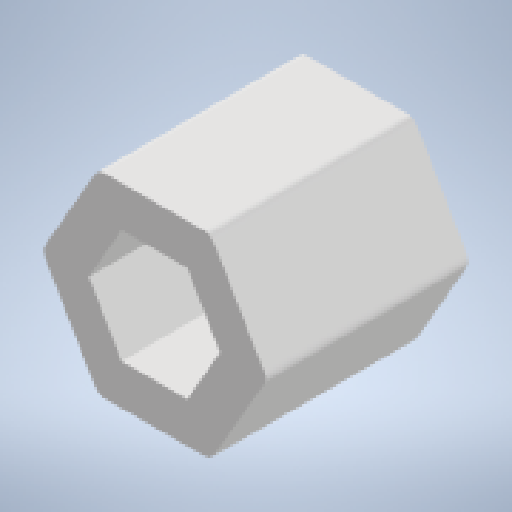
# Autodesk Inventor part: TurretTighteningNut
Saved by Autodesk Inventor 2023 (Build 270158000, 158)
## iProperties
Created: 2023-05-07
Part Number: TurretTighteningNut
Material: Generic
Document SubType Name: Modeling
Designer: karpova
Density: 1 g/cm^3
Appearance: Default
Author: karpova
Autodesk Inventor part; units mm, degrees
ref_plane "YZ Plane" through (0, 0, 0) normal (1, 0, 0) x (0, 1, 0)
ref_plane "XZ Plane" through (0, 0, 0) normal (0, 1, 0) x (-1, 0, 0)
ref_plane "XY Plane" through (0, 0, 0) normal (0, 0, 1) x (1, 0, 0)
sketch "Sketch1" plane through (0, 0, 0) normal (0, 0, 1) x (1, 0, 0)
  circle A0 centre (0.0756, -0.4532) radius 1.5 projected
  circle A1 centre (0.0756, -0.4532) radius 1.7 projected
  circle A2 centre (0.0756, -0.4532) radius 1.7 projected
  circle A3 centre (0.0756, -0.4532) radius 1.8
  line L0 (2.8469, 4.3468) -> (5.6182, -0.4532)
  line L1 (5.6182, -0.4532) -> (2.8469, -5.2532)
  line L2 (2.8469, -5.2532) -> (-2.6957, -5.2532)
  line L3 (-2.6957, -5.2532) -> (-5.4669, -0.4532)
  line L4 (-5.4669, -0.4532) -> (-2.6957, 4.3468)
  line L5 (-2.6957, 4.3468) -> (2.8469, 4.3468)
  line L6 (-1.558, 1.3468) -> (2.6621, 1.3468) construction
  point P0 (0, 0)
  dimension "d0" = 0.1
  dimension "d1" = 3
  constraints: 14 end point, 1 centre point, 1 coincident, 1 horizontal, 1 parallel, 1 tangent, 13 other
  measures "d0" radial gap between concentric circles of A1 A3
  measures "d1" distance between parallel lines of L5 L6
extrude "Extrusion1" add sketch "Sketch1" along normal blind 4 contours L0 L1 L2 L3 L4 L5
sketch "Sketch2" plane through (0, 0, 4) normal (0, 0, 1) x (1, 0, 0)
  line L0 (-2.6957, 4.3468) -> (-5.4669, -0.4532) projected
  line L1 (-5.4669, -0.4532) -> (-2.6957, -5.2532) projected
  line L2 (-2.6957, -5.2532) -> (2.8469, -5.2532) projected
  line L3 (2.8469, -5.2532) -> (5.6182, -0.4532) projected
  line L4 (5.6182, -0.4532) -> (2.8469, 4.3468) projected
  line L5 (2.8469, 4.3468) -> (-2.6957, 4.3468) projected
  circle A0 centre (0.0756, -0.4532) radius 1.8 projected
  line L6 (-3.1575, -0.4532) -> (-1.541, 2.3468)
  line L7 (-1.541, 2.3468) -> (1.6922, 2.3468)
  line L8 (1.6922, 2.3468) -> (3.3088, -0.4532)
  line L9 (3.3088, -0.4532) -> (1.6922, -3.2532)
  line L10 (1.6922, -3.2532) -> (-1.541, -3.2532)
  line L11 (-1.541, -3.2532) -> (-3.1575, -0.4532)
  point P0 (0, 0)
  dimension "d4" = 2
  constraints: 12 end point, 5 other
  measures "d4" distance between parallel lines of L0 L6
extrude "Extrusion2" add sketch "Sketch2" along normal blind 6 contours L5 L4 L3 L2 L1 L0
fillet "Fillet1" radius 0.5 6 edges at (-5.4669, -0.4532, 5) (-2.6957, 4.3468, 5) (2.8469, 4.3468, 5) (5.6182, -0.4532, 5) (-2.6957, -5.2532, 5) (2.8469, -5.2532, 5)
thread "Thread1" size "M3x0.5" class "6H" standard "ANSI Metric M Profile" full length
body "Solid1"
